Axe 6 v2 (Autodesk Fusion 360 design; units mm, degrees)
Autodesk Fusion 360 part; units mm, degrees
sketch "Sketch1" plane through (0, 0, 0) normal (0, 0, 1) x (1, 0, 0)
  circle A0 centre (0, 0) radius 9.5
  circle A1 centre (0, 0) radius 7.5
  line L0 (4.1569, 0) -> (2.0785, 3.6)
  line L1 (2.0785, 3.6) -> (-2.0785, 3.6)
  line L2 (-2.0785, 3.6) -> (-4.1569, 0)
  line L3 (-4.1569, 0) -> (-2.0785, -3.6)
  line L4 (-2.0785, -3.6) -> (2.0785, -3.6)
  line L5 (2.0785, -3.6) -> (4.1569, 0)
  line L6 (-4.1569, 0) -> (4.1569, 0) construction
  dimension "d1" = 19
  dimension "d2" = 15
  dimension "d3" = 7.2
  constraint coincident A0.centre A1.centre
  constraint horizontal L6
  measures "d1" diameter of A0
  measures "d2" diameter of A1
  measures "d3" distance of L2 L5
extrude "Extrude1" add sketch "Sketch1" along normal blind 0.5 contours A1
extrude "Extrude2" [suppressed]
extrude "Extrude3" [suppressed]
named bodies: "Axe 6"
